Autodesk Fusion 360 part; units mm, degrees
(part 2 of 3)
  point P10 (75, -26)
  point P11 (105, -26)
  point P12 (60, 0)
  point P13 (60, 0)
  point P14 (90, 0)
  point P15 (60, 0)
  point P16 (90, 0)
  point P17 (15, -26)
  point P18 (15, -26)
  point P19 (45, -26)
  point P20 (15, -26)
  point P21 (45, -26)
  point P22 (105, -26)
  point P23 (60, 0)
  point P24 (105, -26)
  point P25 (90, 0)
  point P26 (90, 0)
  point P27 (60, 0)
  point P28 (75, -26)
  point P29 (75, -26)
  point P30 (75, -26)
  point P31 (60, 0)
  point P32 (30, 0)
  point P33 (30, 0)
  point P34 (60, -52)
  point P35 (75, -78)
  point P36 (60, -52)
  point P37 (90, -52)
  point P38 (90, -52)
  point P39 (75, -78)
  point P40 (60, -52)
  point P41 (0, -52)
  point P42 (105, -78)
  point P43 (30, -52)
  point P44 (75, -78)
  point P45 (0, -52)
  point P46 (105, -78)
  point P47 (0, -52)
  point P48 (15, -78)
  point P49 (45, -78)
  point P50 (15, -78)
  point P51 (15, -78)
  point P52 (45, -78)
  point P53 (15, -78)
  point P54 (15, -78)
  point P55 (45, -78)
  point P56 (15, -78)
  point P57 (45, -78)
  point P58 (105, -78)
  point P59 (60, -52)
  point P60 (105, -78)
  point P61 (90, -52)
  point P62 (90, -52)
  point P63 (60, -52)
  point P64 (75, -78)
  point P65 (75, -78)
  point P66 (75, -78)
  point P67 (60, -52)
  point P68 (0, -52)
  point P69 (0, -52)
  point P70 (30, -52)
  point P71 (30, -52)
  point P72 (0, -52)
  point P73 (30, -52)
  dimension "d7" = 16
  dimension "d8" = 16
  dimension "d9" = 2
  dimension "d10" = 14.5
  dimension "d11" = 14.5
  dimension "d14" = 16
  dimension "d15" = 16
  dimension "d16" = 2
  dimension "d17" = 14.5
  dimension "d18" = 14.5
  dimension "d19" = 16
  dimension "d20" = 16
  dimension "d21" = 2
  dimension "d22" = 14.5
  dimension "d23" = 14.5
  dimension "d24" = 16
  dimension "d25" = 16
  dimension "d26" = 2
  dimension "d27" = 14.5
  dimension "d28" = 14.5
  dimension "d29" = 16
  dimension "d30" = 16
  dimension "d31" = 2
  dimension "d32" = 14.5
  dimension "d33" = 14.5
  dimension "d34" = 16
  dimension "d35" = 16
  dimension "d36" = 2
  dimension "d37" = 14.5
  dimension "d38" = 14.5
  dimension "d39" = 16
  dimension "d40" = 16
  dimension "d41" = 2
  dimension "d42" = 14.5
  dimension "d43" = 14.5
  dimension "d44" = 16
  dimension "d45" = 16
  dimension "d46" = 2
  dimension "d47" = 14.5
  dimension "d48" = 14.5
  dimension "d49" = 16
  dimension "d50" = 16
  dimension "d51" = 2
  dimension "d52" = 14.5
  dimension "d53" = 14.5
  dimension "d54" = 16
  dimension "d55" = 16
  dimension "d56" = 2
  dimension "d57" = 14.5
  dimension "d58" = 14.5
  dimension "d59" = 16
  dimension "d60" = 16
  dimension "d61" = 2
  dimension "d62" = 14.5
  dimension "d63" = 14.5
  dimension "d64" = 16
  dimension "d65" = 16
  dimension "d66" = 2
  dimension "d67" = 14.5
  dimension "d68" = 14.5
  dimension "d69" = 16
  dimension "d70" = 16
  dimension "d71" = 2
  dimension "d72" = 14.5
  dimension "d73" = 14.5
  dimension "d74" = 16
  dimension "d75" = 16
  dimension "d76" = 2
  dimension "d77" = 14.5
  dimension "d78" = 14.5
  dimension "d79" = 16
  dimension "d80" = 16
  dimension "d81" = 2
  dimension "d82" = 14.5
  dimension "d83" = 14.5
  dimension "d84" = 16
  dimension "d85" = 16
  dimension "d86" = 2
  dimension "d87" = 14.5
  dimension "d88" = 14.5
  constraint coincident P33 P32
  constraint coincident P20 P18
  constraint coincident P21 P19
  constraint coincident P31 P27
  constraint coincident P26 P25
  constraint coincident P30 P29
  constraint coincident P24 P22
  constraint coincident P72 P69
  constraint coincident P73 P71
  constraint coincident P56 P54
  constraint coincident P57 P55
  constraint coincident P67 P63
  constraint coincident P62 P61
  constraint coincident P66 P65
  constraint coincident P60 P58
  measures "d7" distance of origin L5
  measures "d8" distance of P33 L11
  measures "d9" distance of L5 L8
  measures "d10" distance of origin L17
  measures "d11" distance of P33 L23
  measures "d14" distance of P20 L47
  measures "d15" distance of P21 L34
  measures "d16" distance of L27 L47
  measures "d17" distance of P20 L45
  measures "d18" distance of P21 L33
  measures "d19" distance of P31 L77
  measures "d20" distance of P26 L78
  measures "d21" distance of L64 L77
  measures "d22" distance of P31 L61
  measures "d23" distance of P26 L93
  measures "d24" distance of P30 L86
  measures "d25" distance of P24 L88
  measures "d26" distance of L81 L86
  measures "d27" distance of P30 L48
  measures "d28" distance of P24 L55
  measures "d29" distance of origin L137
  measures "d30" distance of P33 L115
  measures "d31" distance of L137 L138
  measures "d32" distance of origin L126
  measures "d33" distance of P33 L116
  measures "d34" distance of P20 L124
  measures "d35" distance of P21 L127
  measures "d36" distance of L124 L140
  measures "d37" distance of P20 L155
  measures "d38" distance of P21 L120
  measures "d39" distance of P31 L185
  measures "d40" distance of P26 L175
  measures "d41" distance of L185 L191
  measures "d42" distance of P31 L170
  measures "d43" distance of P26 L99
  measures "d44" distance of P30 L150
  measures "d45" distance of P24 L147
  measures "d46" distance of L150 L163
  measures "d47" distance of P30 L158
  measures "d48" distance of P24 L151
  measures "d49" distance of P72 L360
  measures "d50" distance of P73 L338
  measures "d51" distance of L309 L360
  measures "d52" distance of P72 L381
  measures "d53" distance of P73 L340
  measures "d54" distance of P56 L319
  measures "d55" distance of P57 L327
  measures "d56" distance of L319 L332
  measures "d57" distance of P56 L275
  measures "d58" distance of P57 L331
  measures "d59" distance of P67 L365
  measures "d60" distance of P62 L375
  measures "d61" distance of L342 L365
  measures "d62" distance of P67 L336
  measures "d63" distance of P62 L352
  measures "d64" distance of P66 L300
  measures "d65" distance of P60 L320
  measures "d66" distance of L274 L300
  measures "d67" distance of P66 L203
  measures "d68" distance of P60 L317
  measures "d69" distance of P72 L369
  measures "d70" distance of P73 L263
  measures "d71" distance of L369 L379
  measures "d72" distance of P72 L358
  measures "d73" distance of P73 L228
  measures "d74" distance of P56 L196
  measures "d75" distance of P57 L214
  measures "d76" distance of L196 L334
  measures "d77" distance of P56 L219
  measures "d78" distance of P57 L292
  measures "d79" distance of P67 L246
  measures "d80" distance of P62 L235
  measures "d81" distance of L221 L246
  measures "d82" distance of P67 L222
  measures "d83" distance of P62 L227
  measures "d84" distance of P66 L212
  measures "d85" distance of P60 L199
  measures "d86" distance of L208 L212
  measures "d87" distance of P66 L205
  measures "d88" distance of P60 L201
extrude "Extrude2" add sketch "Sketch1" along normal blind 100 contours L0 L5 L7 L8 L12 L17 L19 L20 L37 L43 L96 L118 L126 L128 L129 L137 L138 L143 L145 L161 | L0 L5 L6 L7 L18 L19 L74 L94 L96 L101 L107 L118 L129 L133 L137 L181 | L0 L1 L2 L3 L7 L8 L12 L13 L14 L15 L28 L37 L96 L102 L104 L105 L109 L111 L112 L118 L138 L143 L145 L169 | L6 L11 L50 L59 L64 L67 L74 L80 L106 L107 L115 L136 L176 L181 L187 L191 | L6 L11 L18 L23 L31 L38 L59 L65 L74 L94 L101 L107 L115 L116 L130 L133 L136 L139 L179 L181 | L4 L5 L21 L27 L30 L38 L97 L131 L137 L139 L140 L162 | L4 L5 L8 L9 L16 L17 L20 L21 L24 L30 L37 L43 L97 L98 L126 L128 L131 L137 L138 L142 L145 L161 L162 L168 | L9 L10 L21 L22 L27 L30 L35 L38 L42 L43 L45 L47 L117 L119 L124 L128 L131 L139 L140 L141 L142 L148 L155 L162 | L22 L35 L43 L47 L60 L94 L101 L117 L119 L124 L128 L189 | L3 L4 L8 L9 L15 L16 L24 L28 L37 L41 L97 L98 L102 L109 L111 L114 L138 L142 L145 L168 | L3 L4 L28 L41 L97 L102 L111 L114 L237 L265 L266 L345 | L50 L56 L67 L71 L73 L75 L77 L78 L79 L93 L99 L106 L167 L171 L174 L175 L176 L180 L184 L185 | L50 L61 L64 L67 L68 L75 L77 L80 L84 L87 L106 L170 L171 L172 L176 L177 L185 L187 L190 L191 | L10 L11 L22 L23 L25 L31 L35 L38 L60 L65 L92 L94 L101 L115 L116 L117 L119 L123 L130 L139 L141 L179 L183 L189 | L28 L39 L41 L46 L111 L114 L144 L146 L225 L234 L237 L242 L265 L266 L271 L280 L288 L309 L345 L379 | L28 L39 L111 L146 L192 L240 L241 L242 L244 L247 L249 L258 L260 L261 L264 L266 L270 L271 L345 L355 | L10 L11 L25 L66 L87 L92 L115 L123 L141 L153 L183 L190 | L25 L31 L33 L34 L49 L52 L60 L66 L82 L87 L92 L95 L103 L113 L120 L123 L127 L130 L134 L153 L173 L183 L189 L190 | L31 L34 L52 L62 L64 L95 L113 L127 L130 L173 L188 L191 | L56 L57 L58 L71 L72 L76 L78 L84 L86 L93 L99 L100 L110 L150 L174 L175 L177 L178 L180 L186 | L55 L56 L63 L72 L76 L78 L83 L88 L100 L147 L149 L151 L164 L174 L175 L186 L230 L235 L375 L380 | L9 L10 L42 L45 L141 L142 L148 L155 L280 L288 L324 L326 | L198 L204 L218 L220 L224 L226 L238 L241 L245 L247 L252 L254 L260 L264 L269 L290 L299 L301 L332 L334 | L192 L223 L226 L229 L231 L240 L241 L244 L245 L247 L254 L257 L260 L261 L264 L268 L269 L285 L309 L379 | L49 L52 L61 L62 L64 L68 L70 L77 L84 L87 L90 L95 L103 L108 L113 L170 L172 L173 L177 L182 L185 L188 L190 L191 | L49 L70 L71 L77 L81 L90 L103 L108 L163 L180 L182 L185 | L26 L27 L29 L36 L42 L44 L45 L47 L124 L125 L132 L140 L148 L154 L155 L156 L278 L280 L281 L287 L288 L308 L324 L326 | L26 L27 L29 L125 L140 L156 L237 L265 L278 L308 L360 L369 | L36 L44 L47 L124 L132 L154 L248 L267 L281 L287 L339 L362 | L26 L39 L44 L46 L125 L132 L144 L146 L225 L234 L237 L265 L278 L280 L288 L308 L309 L312 L356 L358 L360 L369 L379 L381 | L39 L44 L132 L146 L192 L244 L312 L323 L350 L356 L358 L381 | L48 L57 L58 L62 L70 L71 L76 L81 L84 L85 L86 L90 L100 L108 L110 L150 L158 L163 L165 L177 L178 L180 L182 L188 | L33 L49 L60 L82 L103 L120 L134 L189 L239 L267 L339 L354 | L29 L32 L36 L40 L121 L135 L154 L156 L228 L233 L248 L253 L263 L267 L281 L287 L324 L326 L338 L339 L340 L341 L362 L378 | L32 L51 L66 L121 L153 L160 L253 L263 L324 L326 L338 L341 | L192 L223 L226 L229 L231 L244 L245 L257 L268 L279 L285 L305 L309 L312 L323 L350 L356 L358 L360 L369 L370 L371 L379 L381 | L63 L91 L122 L164 L227 L235 L293 L313 L344 L347 L352 L375 | L53 L63 L69 L83 L86 L91 L122 L149 L150 L152 L157 L164 L227 L230 L235 L255 L352 L375 L377 L380 | L32 L33 L34 L40 L51 L66 L82 L89 L120 L121 L127 L134 L135 L153 L160 L166 L239 L251 L253 L267 L339 L341 L354 L374 | L196 L197 L198 L202 L204 L218 L219 L268 L275 L285 L289 L290 L291 L299 L301 L319 L321 L332 L334 L364 | L193 L196 L198 L200 L202 L204 L215 L273 L282 L283 L290 L291 L301 L319 L325 L328 | L195 L199 L201 L206 L207 L210 L211 L212 L213 L216 L235 L286 L293 L300 L303 L316 L317 L320 L335 L344 L349 L351 L353 L375 | L212 L227 L235 L293 L295 L300 L313 L316 L318 L329 L343 L344 L347 L349 L351 L352 L353 L359 L363 L375 | L48 L62 L76 L85 L100 L158 L165 L188 L230 L236 L346 L380 | L226 L245 L262 L279 L296 L305 L332 L334 L360 L369 L370 L371 | L34 L40 L89 L127 L135 L166 L221 L236 L251 L342 L346 L374 | L48 L53 L54 L69 L81 L85 L86 L91 L122 L150 L152 L157 L158 L159 L163 L165 L230 L232 L236 L255 L346 L357 L377 L380 | L193 L200 L209 L214 L215 L272 L273 L276 L282 L283 L292 L302 L314 L315 L325 L327 L328 L331 L348 L373 | L200 L206 L207 L208 L214 L216 L217 L273 L274 L282 L304 L314 L315 L325 L327 L335 | L196 L197 L219 L259 L262 L268 L275 L279 L285 L289 L296 L305 L307 L310 L319 L321 L323 L332 L334 L350 L361 L364 L370 L371 | L51 L53 L54 L89 L157 L159 L160 L166 L221 L222 L232 L236 L239 L246 L251 L336 L337 L342 L346 L354 L357 L365 L374 L383 | L54 L81 L91 L122 L159 L163 L232 L239 L246 L354 L357 L365 | L29 L40 L135 L156 L228 L233 L262 L294 L296 L340 L372 L378 | L228 L233 L248 L256 L259 L262 L263 L272 L277 L294 L296 L298 L307 L310 L321 L338 L340 L361 L362 L364 L368 L372 L373 L378 | L196 L248 L259 L272 L307 L310 L319 L323 L350 L361 L362 L373 | L193 L250 L256 L263 L277 L283 L298 L306 L321 L338 L364 L368 | L194 L203 L205 L206 L207 L208 L210 L212 L213 L216 L217 L243 L274 L300 L304 L311 L333 L335 L351 L353 | L51 L53 L157 L160 L222 L250 L306 L318 L336 L337 L343 L383 | L194 L203 L205 L208 L212 L243 L274 L295 L297 L300 L311 L313 L318 L322 L329 L333 L343 L347 L351 L353 L359 L363 L366 L376 | L208 L246 L274 L276 L297 L313 L322 L347 L348 L365 L366 L376 | L193 L209 L214 L250 L256 L272 L276 L277 L283 L284 L292 L294 L298 L302 L306 L327 L330 L331 L348 L367 L368 L372 L373 L382 | L214 L221 L243 L284 L294 L311 L327 L330 L342 L367 L372 L382 | L221 L222 L243 L246 L250 L276 L284 L297 L306 L311 L318 L322 L330 L336 L337 L342 L343 L348 L365 L366 L367 L376 L382 L383
extrude "Extrude3" add sketch "Sketch1" along normal blind 3
sketch "Sketch2" plane through (0, 0, 0) normal (1, 0, 0) x (0, 0, -1)
  circle A0 centre (0, 0) radius 100.9277
  line L0 (0, 100.9277) -> (-120.0555, 100.9277)
  line L1 (-100.9261, -0.5759) -> (-100.9261, 117.8677)
  constraint coincident A0.centre origin
  constraint coincident A0 L0.start
  constraint tangent A0 L0
  constraint horizontal L0
  constraint coincident A0 L1.start
  constraint perpendicular L0 L1
extrude "Extrude4" cut sketch "Sketch2" along normal blind 169 and the other way blind 53 contours A0 L0 L1
sketch "Sketch3" plane through (0, 0, 0) normal (0, 1, 0) x (1, 0, 0)
  circle A0 centre (0, 0) radius 1.5
  circle A1 centre (30, 0) radius 1.5
  circle A2 centre (15, -26) radius 1.5
  circle A3 centre (0, -52) radius 1.5
  circle A4 centre (15, -78) radius 1.5
  circle A5 centre (45, -78) radius 1.5
  circle A6 centre (30, -52) radius 1.5
  circle A7 centre (45, -26) radius 1.5
  circle A8 centre (60, 0) radius 1.5
  circle A9 centre (90, 0) radius 1.5
  circle A10 centre (105, -26) radius 1.5
  circle A11 centre (75, -26) radius 1.5
  circle A12 centre (60, -52) radius 1.5
  circle A13 centre (75, -78) radius 1.5
  circle A14 centre (105, -78) radius 1.5
  circle A15 centre (90, -52) radius 1.5
  point P0 (15, -78)
  point P1 (0, -52)
  point P2 (30, -52)
  point P3 (15, -26)
  point P4 (30, 0)
  point P5 (45, -26)
  point P6 (60, 0)
  point P7 (90, 0)
  point P8 (75, -26)
  point P9 (105, -26)
  point P10 (90, -52)
  point P11 (60, -52)
  point P12 (45, -78)
  point P13 (75, -78)
  point P14 (105, -78)
  dimension "d97" = 3
  constraint coincident A0.centre origin
  constraint coincident P4 A1.centre
  constraint coincident P3 A2.centre
  constraint coincident P1 A3.centre
  constraint coincident P0 A4.centre
  constraint coincident P12 A5.centre
  constraint coincident P2 A6.centre
  constraint coincident P5 A7.centre
  constraint coincident P6 A8.centre
  constraint coincident P7 A9.centre
  constraint coincident P9 A10.centre
  constraint coincident P8 A11.centre
  constraint coincident P11 A12.centre
  constraint coincident P13 A13.centre
  constraint coincident P14 A14.centre
  constraint coincident P10 A15.centre
  constraint equal A4 A5
  constraint equal A5 A13
  constraint equal A13 A14
  constraint equal A3 A14
  constraint equal A3 A6
  constraint equal A6 A12
  constraint equal A12 A15
  constraint equal A2 A15
  constraint equal A2 A7
  constraint equal A7 A11
  constraint equal A10 A11
  constraint equal A0 A10
  constraint equal A0 A1
  constraint equal A1 A8
  constraint equal A8 A9
  measures "d97" diameter of A0
equation "d7 = size1"
equation "d8 = size1"
equation "d10 = size2"
equation "d11 = size2"
equation "d14 = size1"
equation "d17 = size2"
equation "d18 = size2"
equation "d19 = size1"
equation "d20 = size1"
equation "d22 = size2"
equation "d23 = size2"
equation "d24 = size1"
equation "d25 = size1"
equation "d27 = size2"
equation "d28 = size2"
equation "d29 = size1"
equation "d30 = size1"
equation "d32 = size2"
equation "d33 = size2"
equation "d34 = size1"
equation "d37 = size2"
equation "d38 = size2"
equation "d39 = size1"
equation "d40 = size1"
equation "d42 = size2"
equation "d43 = size2"
equation "d44 = size1"
equation "d45 = size1"
equation "d47 = size2"
equation "d48 = size2"
equation "d49 = size1"
equation "d50 = size1"
equation "d52 = size2"
equation "d53 = size2"
equation "d54 = size1"
equation "d55 = size1"
equation "d57 = size2"
equation "d58 = size2"
equation "d59 = size1"
equation "d60 = size1"
equation "d62 = size2"
equation "d63 = size2"
equation "d64 = size1"
equation "d65 = size1"
equation "d67 = size2"
equation "d68 = size2"
equation "d69 = size1"
equation "d70 = size1"
equation "d72 = size2"
equation "d73 = size2"
equation "d74 = size1"
equation "d77 = size2"
equation "d78 = size2"
equation "d79 = size1"
equation "d80 = size1"
equation "d82 = size2"
equation "d83 = size2"
equation "d84 = size1"
equation "d85 = size1"
equation "d87 = size2"
equation "d88 = size2"
equation "size1 = 16 mm"
equation "size2 = 14.5 mm"

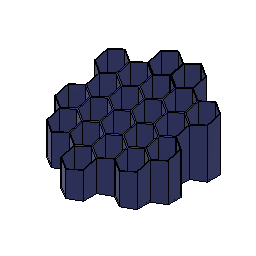
design "hexagon-06"
Autodesk Fusion 360 part; units mm, degrees
sketch "Sketch1" plane through (0, 0, 0) normal (0, 1, 0) x (1, 0, 0)
  line L0 (15.0321, 8.6045) -> (0.0644, 17.3204)
  line L1 (0.0644, 17.3204) -> (-14.9677, 8.7159)
  line L2 (-14.9677, 8.7159) -> (-15.0321, -8.6045)
  line L3 (-15.0321, -8.6045) -> (-0.0644, -17.3204)
  line L4 (-0.0644, -17.3204) -> (14.9677, -8.7159)
  line L5 (14.9677, -8.7159) -> (15.0321, 8.6045)
  line L6 (14.9677, -8.7159) -> (-0.0644, -17.3204)
  line L7 (-0.0644, -17.3204) -> (-0.1287, -34.6408)
  line L8 (-0.1287, -34.6408) -> (14.839, -43.3567)
  line L9 (14.839, -43.3567) -> (29.8711, -34.7523)
  line L10 (29.8711, -34.7523) -> (29.9354, -17.4319)
  line L11 (29.9354, -17.4319) -> (14.9677, -8.7159)
  line L12 (14.839, -43.3567) -> (-0.1287, -34.6408)
  line L13 (-0.1287, -34.6408) -> (-15.1608, -43.2452)
  line L14 (-15.1608, -43.2452) -> (-15.2252, -60.5656)
  line L15 (-15.2252, -60.5656) -> (-0.2575, -69.2816)
  line L16 (-0.2575, -69.2816) -> (14.7746, -60.6771)
  line L17 (14.7746, -60.6771) -> (14.839, -43.3567)
  line L18 (14.2, 8.1984) -> (0, 16.3967)
  line L19 (0, 16.3967) -> (-14.2, 8.1984)
  line L20 (-14.2, 8.1984) -> (-14.2, -8.1984)
  line L21 (-14.2, -8.1984) -> (0, -16.3967)
  line L22 (0, -16.3967) -> (14.2, -8.1984)
  line L23 (14.2, -8.1984) -> (14.2, 8.1984)
  line L24 (29.1033, -17.838) -> (14.9033, -9.6396)
  line L25 (14.9033, -9.6396) -> (0.7033, -17.838)
  line L26 (0.7033, -17.838) -> (0.7033, -34.2347)
  line L27 (0.7033, -34.2347) -> (14.9033, -42.4331)
  line L28 (14.9033, -42.4331) -> (29.1033, -34.2347)
  line L29 (29.1033, -34.2347) -> (29.1033, -17.838)
  line L30 (14.0069, -43.7628) -> (-0.1931, -35.5644)
  line L31 (-0.1931, -35.5644) -> (-14.3931, -43.7628)
  line L32 (-14.3931, -43.7628) -> (-14.3931, -60.1595)
  line L33 (-14.3931, -60.1595) -> (-0.1931, -68.3579)
  line L34 (-0.1931, -68.3579) -> (14.0069, -60.1595)
  line L35 (14.0069, -60.1595) -> (14.0069, -43.7628)
  line L36 (14.7746, -60.6771) -> (-0.2575, -69.2816)
  line L37 (-0.2575, -69.2816) -> (-0.3218, -86.6019)
  line L38 (-0.3218, -86.6019) -> (14.6459, -95.3179)
  line L39 (14.6459, -95.3179) -> (29.678, -86.7134)
  line L40 (29.678, -86.7134) -> (29.7423, -69.393)
  line L41 (29.7423, -69.393) -> (14.7746, -60.6771)
  line L42 (28.9103, -69.7991) -> (14.7103, -61.6007)
  line L43 (14.7103, -61.6007) -> (0.5103, -69.7991)
  line L44 (0.5103, -69.7991) -> (0.5103, -86.1959)
  line L45 (0.5103, -86.1959) -> (14.7103, -94.3942)
  line L46 (14.7103, -94.3942) -> (28.9103, -86.1959)
  line L47 (28.9103, -86.1959) -> (28.9103, -69.7991)
  line L48 (44.7746, -60.6771) -> (29.7425, -69.2816)
  line L49 (44.9677, -8.7159) -> (45.0321, 8.6045)
  line L50 (44.9033, -9.6396) -> (30.7033, -17.838)
  line L51 (29.9356, -17.3204) -> (44.9677, -8.7159)
  line L52 (15.8, 8.1984) -> (15.8, -8.1984)
  line L53 (14.7748, -60.5656) -> (29.7425, -69.2816)
  line L54 (30, -16.3967) -> (44.2, -8.1984)
  line L55 (29.7425, -69.2816) -> (29.6782, -86.6019)
  line L56 (44.7103, -61.6007) -> (30.5103, -69.7991)
  line L57 (29.8069, -68.3579) -> (44.0069, -60.1595)
  line L58 (45.0321, 8.6045) -> (30.0644, 17.3204)
  line L59 (15.0323, 8.7159) -> (14.9679, -8.6045)
  line L60 (30.5103, -69.7991) -> (30.5103, -86.1959)
  line L61 (30.7033, -17.838) -> (30.7033, -34.2347)
  line L62 (29.8713, -34.6408) -> (14.8392, -43.2452)
  line L63 (15.8, -8.1984) -> (30, -16.3967)
  line L64 (30, 16.3967) -> (15.8, 8.1984)
  line L65 (29.8069, -35.5644) -> (15.6069, -43.7628)
  line L66 (44.839, -43.3567) -> (29.8713, -34.6408)
  line L67 (30.0644, 17.3204) -> (15.0323, 8.7159)
  line L68 (44.0069, -43.7628) -> (29.8069, -35.5644)
  line L69 (29.9356, -17.3204) -> (29.8713, -34.6408)
  line L70 (44.2, -8.1984) -> (44.2, 8.1984)
  line L71 (30.7033, -34.2347) -> (44.9033, -42.4331)
  line L72 (44.9677, -8.7159) -> (29.9356, -17.3204)
  line L73 (44.2, 8.1984) -> (30, 16.3967)
  line L74 (58.9103, -69.7991) -> (44.7103, -61.6007)
  line L75 (59.9354, -17.4319) -> (44.9677, -8.7159)
  line L76 (59.7423, -69.393) -> (44.7746, -60.6771)
  line L77 (44.9033, -42.4331) -> (59.1033, -34.2347)
  line L78 (59.678, -86.7134) -> (59.7423, -69.393)
  line L79 (59.1033, -17.838) -> (44.9033, -9.6396)
  line L80 (44.6459, -95.3179) -> (59.678, -86.7134)
  line L81 (44.839, -43.3567) -> (59.8711, -34.7523)
  line L82 (59.8711, -34.7523) -> (59.9354, -17.4319)
  line L83 (59.1033, -34.2347) -> (59.1033, -17.838)
  line L84 (15.6069, -60.1595) -> (29.8069, -68.3579)
  line L85 (44.0069, -60.1595) -> (44.0069, -43.7628)
  line L86 (29.6782, -86.6019) -> (44.6459, -95.3179)
  line L87 (30.5103, -86.1959) -> (44.7103, -94.3942)
  line L88 (14.9679, -8.6045) -> (29.9356, -17.3204)
  line L89 (29.7425, -69.2816) -> (44.7746, -60.6771)
  line L90 (29.8713, -34.6408) -> (44.839, -43.3567)
  line L91 (58.9103, -86.1959) -> (58.9103, -69.7991)
  line L92 (44.7103, -94.3942) -> (58.9103, -86.1959)
  line L93 (44.7746, -60.6771) -> (44.839, -43.3567)
  line L94 (14.8392, -43.2452) -> (14.7748, -60.5656)
  line L95 (15.6069, -43.7628) -> (15.6069, -60.1595)
  line L96 (74.7746, -60.6771) -> (59.7425, -69.2816)
  line L97 (74.9677, -8.7159) -> (75.0321, 8.6045)
  line L98 (74.9033, -9.6396) -> (60.7033, -17.838)
  line L99 (59.9356, -17.3204) -> (74.9677, -8.7159)
  line L100 (45.8, 8.1984) -> (45.8, -8.1984)
  line L101 (44.7748, -60.5656) -> (59.7425, -69.2816)
  line L102 (60, -16.3967) -> (74.2, -8.1984)
  line L103 (59.7425, -69.2816) -> (59.6782, -86.6019)
  line L104 (74.7103, -61.6007) -> (60.5103, -69.7991)
  line L105 (59.8069, -68.3579) -> (74.0069, -60.1595)
  line L106 (75.0321, 8.6045) -> (60.0644, 17.3204)
  line L107 (45.0323, 8.7159) -> (44.9679, -8.6045)
  line L108 (60.5103, -69.7991) -> (60.5103, -86.1959)
  line L109 (60.7033, -17.838) -> (60.7033, -34.2347)
  line L110 (59.8713, -34.6408) -> (44.8392, -43.2452)
  line L111 (45.8, -8.1984) -> (60, -16.3967)
  line L112 (60, 16.3967) -> (45.8, 8.1984)
  line L113 (59.8069, -35.5644) -> (45.6069, -43.7628)
  line L114 (74.839, -43.3567) -> (59.8713, -34.6408)
  line L115 (60.0644, 17.3204) -> (45.0323, 8.7159)
  line L116 (74.0069, -43.7628) -> (59.8069, -35.5644)
  line L117 (59.9356, -17.3204) -> (59.8713, -34.6408)
  line L118 (74.2, -8.1984) -> (74.2, 8.1984)
  line L119 (60.7033, -34.2347) -> (74.9033, -42.4331)
  line L120 (74.9677, -8.7159) -> (59.9356, -17.3204)
  line L121 (74.2, 8.1984) -> (60, 16.3967)
  line L122 (88.9103, -69.7991) -> (74.7103, -61.6007)
  line L123 (89.9354, -17.4319) -> (74.9677, -8.7159)
  line L124 (89.7423, -69.393) -> (74.7746, -60.6771)
  line L125 (74.9033, -42.4331) -> (89.1033, -34.2347)
  line L126 (89.678, -86.7134) -> (89.7423, -69.393)
  line L127 (89.1033, -17.838) -> (74.9033, -9.6396)
  line L128 (74.6459, -95.3179) -> (89.678, -86.7134)
  line L129 (74.839, -43.3567) -> (89.8711, -34.7523)
  line L130 (89.8711, -34.7523) -> (89.9354, -17.4319)
  line L131 (89.1033, -34.2347) -> (89.1033, -17.838)
  line L132 (45.6069, -60.1595) -> (59.8069, -68.3579)
  line L133 (74.0069, -60.1595) -> (74.0069, -43.7628)
  line L134 (59.6782, -86.6019) -> (74.6459, -95.3179)
  line L135 (60.5103, -86.1959) -> (74.7103, -94.3942)
  line L136 (44.9679, -8.6045) -> (59.9356, -17.3204)
  line L137 (59.7425, -69.2816) -> (74.7746, -60.6771)
  line L138 (59.8713, -34.6408) -> (74.839, -43.3567)
  line L139 (88.9103, -86.1959) -> (88.9103, -69.7991)
  line L140 (74.7103, -94.3942) -> (88.9103, -86.1959)
  line L141 (74.7746, -60.6771) -> (74.839, -43.3567)
  line L142 (44.8392, -43.2452) -> (44.7748, -60.5656)
  line L143 (45.6069, -43.7628) -> (45.6069, -60.1595)
  line L144 (104.7746, -60.6771) -> (89.7425, -69.2816)
  line L145 (104.9677, -8.7159) -> (105.0321, 8.6045)
  line L146 (104.9033, -9.6396) -> (90.7033, -17.838)
  line L147 (89.9356, -17.3204) -> (104.9677, -8.7159)
  line L148 (75.8, 8.1984) -> (75.8, -8.1984)
  line L149 (74.7748, -60.5656) -> (89.7425, -69.2816)
  line L150 (90, -16.3967) -> (104.2, -8.1984)
  line L151 (89.7425, -69.2816) -> (89.6782, -86.6019)
  line L152 (104.7103, -61.6007) -> (90.5103, -69.7991)
  line L153 (89.8069, -68.3579) -> (104.0069, -60.1595)
  line L154 (105.0321, 8.6045) -> (90.0644, 17.3204)
  line L155 (75.0323, 8.7159) -> (74.9679, -8.6045)
  line L156 (90.5103, -69.7991) -> (90.5103, -86.1959)
  line L157 (90.7033, -17.838) -> (90.7033, -34.2347)
  line L158 (89.8713, -34.6408) -> (74.8392, -43.2452)
  line L159 (75.8, -8.1984) -> (90, -16.3967)
  line L160 (90, 16.3967) -> (75.8, 8.1984)
  line L161 (89.8069, -35.5644) -> (75.6069, -43.7628)
  line L162 (104.839, -43.3567) -> (89.8713, -34.6408)
  line L163 (90.0644, 17.3204) -> (75.0323, 8.7159)
  line L164 (104.0069, -43.7628) -> (89.8069, -35.5644)
  line L165 (89.9356, -17.3204) -> (89.8713, -34.6408)
  line L166 (104.2, -8.1984) -> (104.2, 8.1984)
  line L167 (90.7033, -34.2347) -> (104.9033, -42.4331)
  line L168 (104.9677, -8.7159) -> (89.9356, -17.3204)
  line L169 (104.2, 8.1984) -> (90, 16.3967)
  line L170 (118.9103, -69.7991) -> (104.7103, -61.6007)
  line L171 (119.9354, -17.4319) -> (104.9677, -8.7159)
  line L172 (119.7423, -69.393) -> (104.7746, -60.6771)
  line L173 (104.9033, -42.4331) -> (119.1033, -34.2347)
  line L174 (119.678, -86.7134) -> (119.7423, -69.393)
  line L175 (119.1033, -17.838) -> (104.9033, -9.6396)
  line L176 (104.6459, -95.3179) -> (119.678, -86.7134)
  line L177 (104.839, -43.3567) -> (119.8711, -34.7523)
  line L178 (119.8711, -34.7523) -> (119.9354, -17.4319)
  line L179 (119.1033, -34.2347) -> (119.1033, -17.838)
  line L180 (75.6069, -60.1595) -> (89.8069, -68.3579)
  line L181 (104.0069, -60.1595) -> (104.0069, -43.7628)
  line L182 (89.6782, -86.6019) -> (104.6459, -95.3179)
  line L183 (90.5103, -86.1959) -> (104.7103, -94.3942)
  line L184 (74.9679, -8.6045) -> (89.9356, -17.3204)
  line L185 (89.7425, -69.2816) -> (104.7746, -60.6771)
  line L186 (89.8713, -34.6408) -> (104.839, -43.3567)
  line L187 (118.9103, -86.1959) -> (118.9103, -69.7991)
  line L188 (104.7103, -94.3942) -> (118.9103, -86.1959)
  line L189 (104.7746, -60.6771) -> (104.839, -43.3567)
  line L190 (74.8392, -43.2452) -> (74.7748, -60.5656)
  line L191 (75.6069, -43.7628) -> (75.6069, -60.1595)
  line L192 (30.0644, 17.3204) -> (45.0323, 8.7159)
  line L193 (45.0323, 8.7159) -> (59.9679, 17.3763)
  line L194 (59.9679, 17.3763) -> (59.9356, 34.6411)
  line L195 (59.9356, 34.6411) -> (44.9677, 43.2456)
  line L196 (44.9677, 43.2456) -> (30.0321, 34.5852)
  line L197 (30.0321, 34.5852) -> (30.0644, 17.3204)
  line L198 (59.9679, 17.3763) -> (75.0323, 8.7159)
  line L199 (75.0323, 8.7159) -> (90.0646, 17.4319)
  line L200 (90.0646, 17.4319) -> (90.0325, 34.8082)
  line L201 (90.0325, 34.8082) -> (74.9681, 43.4686)
  line L202 (74.9681, 43.4686) -> (59.9358, 34.7526)
  line L203 (59.9358, 34.7526) -> (59.9679, 17.3763)
  line L204 (104.9677, -8.7159) -> (119.9354, -17.4319)
  line L205 (119.9354, -17.4319) -> (134.9675, -8.8274)
  line L206 (134.9675, -8.8274) -> (135.0319, 8.493)
  line L207 (135.0319, 8.493) -> (120.0642, 17.2089)
  line L208 (120.0642, 17.2089) -> (105.0321, 8.6045)
  line L209 (105.0321, 8.6045) -> (104.9677, -8.7159)
  line L210 (104.839, -43.3567) -> (104.7746, -60.6771)
  line L211 (104.7746, -60.6771) -> (119.7423, -69.393)
  line L212 (119.7423, -69.393) -> (134.7744, -60.7886)
  line L213 (134.7744, -60.7886) -> (134.8388, -43.4682)
  line L214 (134.8388, -43.4682) -> (119.8711, -34.7523)
  line L215 (119.8711, -34.7523) -> (104.839, -43.3567)
  line L216 (44.6459, -95.3179) -> (44.678, -112.6942)
  line L217 (44.678, -112.6942) -> (59.7423, -121.3546)
  line L218 (59.7423, -121.3546) -> (74.7746, -112.6386)
  line L219 (74.7746, -112.6386) -> (74.7425, -95.2623)
  line L220 (74.7425, -95.2623) -> (59.6782, -86.6019)
  line L221 (59.6782, -86.6019) -> (44.6459, -95.3179)
  line L222 (59.2161, 34.1512) -> (45.0323, 42.3775)
  line L223 (45.0323, 42.3775) -> (30.8162, 34.2071)
  line L224 (30.8162, 34.2071) -> (30.7839, 17.8104)
  line L225 (30.7839, 17.8104) -> (44.9677, 9.584)
  line L226 (44.9677, 9.584) -> (59.1838, 17.7544)
  line L227 (59.1838, 17.7544) -> (59.2161, 34.1512)
  line L228 (89.2002, 34.2906) -> (75.0002, 42.489)
  line L229 (75.0002, 42.489) -> (60.8002, 34.2906)
  line L230 (60.8002, 34.2906) -> (60.8002, 17.8939)
  line L231 (60.8002, 17.8939) -> (75.0002, 9.6955)
  line L232 (75.0002, 9.6955) -> (89.2002, 17.8939)
  line L233 (89.2002, 17.8939) -> (89.2002, 34.2906)
  line L234 (134.0371, -43.9271) -> (119.8676, -35.676)
  line L235 (119.8676, -35.676) -> (105.6373, -43.8216)
  line L236 (105.6373, -43.8216) -> (105.5763, -60.2182)
  line L237 (105.5763, -60.2182) -> (119.7458, -68.4693)
  line L238 (119.7458, -68.4693) -> (133.9761, -60.3237)
  line L239 (133.9761, -60.3237) -> (134.0371, -43.9271)
  line L240 (134.2302, 8.0341) -> (120.0607, 16.2852)
  line L241 (120.0607, 16.2852) -> (105.8304, 8.1396)
  line L242 (105.8304, 8.1396) -> (105.7694, -8.257)
  line L243 (105.7694, -8.257) -> (119.9389, -16.5081)
  line L244 (119.9389, -16.5081) -> (134.1692, -8.3626)
  line L245 (134.1692, -8.3626) -> (134.2302, 8.0341)
  line L246 (73.8951, -95.7537) -> (59.68, -87.5815)
  line L247 (59.68, -87.5815) -> (45.4951, -95.8061)
  line L248 (45.4951, -95.8061) -> (45.5254, -112.2028)
  line L249 (45.5254, -112.2028) -> (59.7405, -120.375)
  line L250 (59.7405, -120.375) -> (73.9254, -112.1504)
  line L251 (73.9254, -112.1504) -> (73.8951, -95.7537)
  point P0 (14.9033, -26.0363)
  point P1 (-0.1931, -51.9612)
  point P2 (14.9033, -26.0363)
  point P3 (-0.1931, -51.9612)
  point P4 (14.7103, -77.9975)
  point P5 (14.7103, -77.9975)
  point P6 (44.9033, -26.0363)
  point P7 (29.8069, -51.9612)
  point P8 (44.9033, -26.0363)
  point P9 (30, 0)
  point P10 (30, 0)
  point P11 (29.8069, -51.9612)
  point P12 (44.7103, -77.9975)
  point P13 (30, 0)
  point P14 (44.7103, -77.9975)
  point P15 (74.9033, -26.0363)
  point P16 (59.8069, -51.9612)
  point P17 (74.9033, -26.0363)
  point P18 (60, 0)
  point P19 (60, 0)
  point P20 (59.8069, -51.9612)
  point P21 (74.7103, -77.9975)
  point P22 (60, 0)
  point P23 (74.7103, -77.9975)
  point P24 (104.9033, -26.0363)
  point P25 (89.8069, -51.9612)
  point P26 (104.9033, -26.0363)
  point P27 (90, 0)
  point P28 (90, 0)
  point P29 (89.8069, -51.9612)
  point P30 (104.7103, -77.9975)
  point P31 (90, 0)
  point P32 (104.7103, -77.9975)
  point P33 (59.8713, -34.6408)
  point P34 (45, 25.9808)
  point P35 (75.0002, 26.0922)
  point P36 (119.9998, -0.1115)
  point P37 (119.8067, -52.0726)
  point P38 (59.7103, -103.9783)
  point P39 (45, 25.9808)
  point P40 (75.0002, 26.0922)
  point P41 (119.8067, -52.0726)
  point P42 (119.9998, -0.1115)
  point P43 (59.7103, -103.9783)
  dimension "d29" = 15
  dimension "d30" = 14.2
  dimension "d31" = 14.2
  dimension "d32" = 14.2
  dimension "d33" = 14.2
  dimension "d36" = 90
  dimension "d37" = 0
  dimension "d47" = 14.2
  dimension "d48" = 14.2
  dimension "d49" = 14.2
  dimension "d50" = 14.2
  dimension "d51" = 14.2
  constraint coincident P2 P0
  constraint coincident P3 P1
  constraint coincident P5 P4
  constraint coincident P33 L110.start
  constraint coincident P39 P34
  constraint coincident P40 P35
  constraint coincident P41 P37
  constraint coincident P42 P36
  constraint coincident P43 P38
  measures "d29" distance of origin L5
  measures "d30" distance of origin L23
  measures "d31" distance of P2 L29
  measures "d32" distance of P3 L35
  measures "d33" distance of P5 L47
  measures "d47" distance of P39 L227
  measures "d48" distance of P40 L233
  measures "d49" distance of P41 L239
  measures "d50" distance of P42 L245
  measures "d51" distance of P43 L251
extrude "Extrude2" add sketch "Sketch1" along normal blind 1.6 contours L0 L5 L59 L88 | L0 L5 L49 L51 L58 L59 L67 L72 L88 L107 L136 | L0 L1 L2 L3 L4 L5 L6 L59 L88 | L5 L11 L69 L88 | L4 L6 L7 L8 L11 L12 L62 L69 L94 | L10 L11 L51 L66 L69 L72 L75 L90 L110 L117 L142 | L192 L193 L194 L195 L196 L197 | L10 L11 L66 L69 L90 | L49 L75 L117 L136 | L49 L58 L97 L99 L106 L107 L115 L120 L136 L155 L184 | L49 L58 L107 L136 | L8 L12 L13 L14 L15 L16 L17 L36 L53 L94 | L8 L9 L10 L12 L62 L66 L90 L94 | L75 L82 L99 L114 L117 L120 L123 L138 L158 L165 L190 | L75 L82 L114 L117 L138 | L198 L199 L200 L201 L202 L203 | L8 L12 L17 L53 L94 | L9 L10 L17 L48 L53 L66 L89 L90 L93 L101 L142 | L66 L81 L82 L90 L110 L114 L138 L142 | L97 L106 L145 L147 L154 L155 L163 L168 L184 L209 | L97 L106 L155 L184 | L66 L90 L93 L101 L142 | L97 L123 L165 L184 | L81 L82 L93 L96 L101 L114 L137 L138 L141 L149 L190 | L17 L41 L53 L55 | L16 L36 L37 L38 L39 L40 L41 L55 L86 | L123 L130 L147 L162 L165 L168 L171 L177 L178 L186 L204 L215 | L123 L130 L162 L165 L186 | L114 L129 L130 L138 L158 L162 L186 L190 | L114 L138 L141 L149 L190 | L145 L171 L204 L205 L206 L207 L208 L209 | L40 L41 L48 L55 L76 L86 L89 L103 L221 | L76 L93 L101 L103 | L129 L130 L141 L144 L149 L162 L185 L186 L189 L210 | L40 L41 L55 L86 | L76 L78 L96 L103 L124 L126 L128 L137 L151 L182 L219 L220 | L124 L141 L149 L151 | L76 L78 L103 L134 L220 | L172 L177 L189 L210 L211 L212 L213 L214 L215 | L124 L126 L144 L151 L172 L174 L176 L182 L185 L211 | L78 L80 L134 L220 L221 | L124 L126 L151 L182 | L78 L80 L128 L134 L216 L217 L218 L219 | L128 L134 L219 L220 | L18 L19 L20 L21 L22 L23 | L24 L25 L26 L27 L28 L29 | L30 L31 L32 L33 L34 L35 | L42 L43 L44 L45 L46 L47 | L50 L61 L71 L77 L79 L83 | L52 L54 L63 L64 L70 L73 | L56 L60 L74 L87 L91 L92 | L57 L65 L68 L84 L85 L95 | L98 L109 L119 L125 L127 L131 | L100 L102 L111 L112 L118 L121 | L104 L108 L122 L135 L139 L140 | L105 L113 L116 L132 L133 L143 | L146 L157 L167 L173 L175 L179 | L148 L150 L159 L160 L166 L169 | L152 L156 L170 L183 L187 L188 | L153 L161 L164 L180 L181 L191 | L222 L223 L224 L225 L226 L227 | L228 L229 L230 L231 L232 L233 | L234 L235 L236 L237 L238 L239 | L240 L241 L242 L243 L244 L245 | L246 L247 L248 L249 L250 L251 makes body 1
extrude "Extrude3" add sketch "Sketch1" along normal blind 80 contours L0 L5 L59 L88 | L0 L5 L49 L51 L58 L59 L67 L72 L88 L107 L136 | L0 L1 L2 L3 L4 L5 L6 L59 L88 | L5 L11 L69 L88 | L4 L6 L7 L8 L11 L12 L62 L69 L94 | L10 L11 L51 L66 L69 L72 L75 L90 L110 L117 L142 | L192 L193 L194 L195 L196 L197 | L10 L11 L66 L69 L90 | L49 L75 L117 L136 | L49 L58 L97 L99 L106 L107 L115 L120 L136 L155 L184 | L49 L58 L107 L136 | L8 L12 L13 L14 L15 L16 L17 L36 L53 L94 | L8 L9 L10 L12 L62 L66 L90 L94 | L75 L82 L99 L114 L117 L120 L123 L138 L158 L165 L190 | L75 L82 L114 L117 L138 | L198 L199 L200 L201 L202 L203 | L8 L12 L17 L53 L94 | L9 L10 L17 L48 L53 L66 L89 L90 L93 L101 L142 | L66 L81 L82 L90 L110 L114 L138 L142 | L97 L106 L145 L147 L154 L155 L163 L168 L184 L209 | L97 L106 L155 L184 | L66 L90 L93 L101 L142 | L97 L123 L165 L184 | L81 L82 L93 L96 L101 L114 L137 L138 L141 L149 L190 | L17 L41 L53 L55 | L16 L36 L37 L38 L39 L40 L41 L55 L86 | L123 L130 L147 L162 L165 L168 L171 L177 L178 L186 L204 L215 | L123 L130 L162 L165 L186 | L114 L129 L130 L138 L158 L162 L186 L190 | L114 L138 L141 L149 L190 | L145 L171 L204 L205 L206 L207 L208 L209 | L40 L41 L48 L55 L76 L86 L89 L103 L221 | L76 L93 L101 L103 | L129 L130 L141 L144 L149 L162 L185 L186 L189 L210 | L40 L41 L55 L86 | L76 L78 L96 L103 L124 L126 L128 L137 L151 L182 L219 L220 | L124 L141 L149 L151 | L76 L78 L103 L134 L220 | L172 L177 L189 L210 L211 L212 L213 L214 L215 | L124 L126 L144 L151 L172 L174 L176 L182 L185 L211 | L78 L80 L134 L220 L221 | L124 L126 L151 L182 | L78 L80 L128 L134 L216 L217 L218 L219 | L128 L134 L219 L220 bodies 1
sketch "Sketch2" plane through (0, 0, 0) normal (1, 0, 0) x (0, 0, -1)
  line L0 (58.2994, 83.577) -> (-124.7141, 32.2408)
  line L1 (-124.7141, 32.2408) -> (-124.7141, 83.577)
  line L2 (-124.7141, 83.577) -> (58.2994, 83.577)
  constraint vertical L1
  constraint perpendicular L1 L2
extrude "Extrude4" cut sketch "Sketch2" along normal blind 159 and the other way blind 41 bodies 1
copy_body "Body->Comp1" bodies 1 removing the originals makes body 2 in component "hexagon-06"
component "hexagon-06" placed x (1, 0, 0) y (0, 1, 0) z (0, 0, 1) at (0, 0, 0)
equation "size1 = 15 mm"
equation "offset1 = 0.8 mm"
equation "d29 = size1"
equation "d30 = size1 - offset1"
equation "d31 = size1 - offset1"
equation "d32 = size1 - offset1"
equation "d33 = size1 - offset1"
equation "d36 = 6 * size1"
equation "d38 = 2 * offset1"
equation "d40 = height"
equation "height = 80 mm"
equation "d47 = size1 - offset1"
equation "d48 = size1 - offset1"
equation "d49 = size1 - offset1"
equation "d50 = size1 - offset1"
equation "d51 = size1 - offset1"

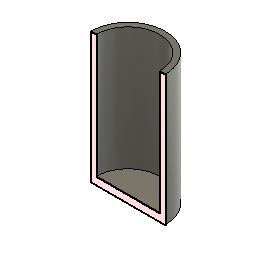
design "tubeToolHolder02"
Autodesk Fusion 360 part; units mm, degrees
sketch "Sketch1" plane through (0, 0, 0) normal (0, 1, 0) x (1, 0, 0)
  circle A0 centre (0, 0) radius 20
  circle A1 centre (0, 0) radius 17
  dimension "d1" = 40
  dimension "d7" = 3
  constraint coincident A0.centre A1.centre
  measures "d1" diameter of A0
  measures "d7" distance of A0 A1
extrude "Extrude1" add sketch "Sketch1" along normal blind 70 makes body 1
extrude "Extrude2" add sketch "Sketch1" along normal blind 4 contours A1 bodies 1
copy_body "Body->Comp1" bodies 1 removing the originals makes body 2 in component "tubeToolHolder02"
component "tubeToolHolder02" placed x (1, 0, 0) y (0, 1, 0) z (0, 0, 1) at (0, 0, 0)

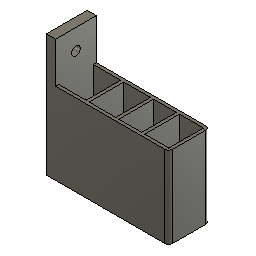
design "item40ToolHolder01"
Autodesk Fusion 360 part; units mm, degrees
sketch "Sketch1" plane through (0, 0, 0) normal (0, 1, 0) x (1, 0, 0)
  line L0 (60, 20) -> (-60, 20)
  line L1 (-60, 20) -> (-60, -20)
  line L2 (-60, -20) -> (60, -20)
  line L3 (60, -20) -> (60, 20)
  line L4 (60, 20) -> (-60, -20) construction
  line L5 (-60, 20) -> (60, -20) construction
  line L6 (57, 17) -> (-57, 17)
  line L7 (-57, 17) -> (-57, -17)
  line L8 (-57, -17) -> (57, -17)
  line L9 (57, -17) -> (57, 17)
  line L10 (57, 17) -> (-57, -17) construction
  line L11 (-57, 17) -> (57, -17) construction
  line L12 (-24.159, 17) -> (-21.159, 17)
  line L13 (-21.159, 17) -> (-21.159, -17)
  line L14 (-21.159, -17) -> (-24.159, -17)
  line L15 (-24.159, -17) -> (-24.159, 17)
  line L16 (8.0431, 17) -> (8.0431, -17)
  line L17 (5.0431, -17) -> (5.0431, 17)
  line L18 (8.0431, -17) -> (5.0431, -17)
  line L19 (5.0431, 17) -> (8.0431, 17)
  line L20 (30.4518, 17) -> (33.4518, 17)
  line L21 (33.4518, 17) -> (33.4518, -17)
  line L22 (30.4518, -17) -> (30.4518, 17)
  line L23 (33.4518, -17) -> (30.4518, -17)
  dimension "d1" = 120
  dimension "d2" = 40
  dimension "d3" = 114
  dimension "d4" = 34
  dimension "d20" = 3
  dimension "d21" = 34
  dimension "d26" = 3
  dimension "d27" = 34
  dimension "d28" = 3
  dimension "d29" = 34
  constraint horizontal L0
  constraint perpendicular L0 L1
  constraint parallel L0 L2
  constraint parallel L1 L3
  constraint coincident L4 origin
  constraint coincident L5 origin
  constraint horizontal L6
  constraint perpendicular L6 L7
  constraint parallel L6 L8
  constraint parallel L7 L9
  constraint coincident L10 origin
  constraint coincident L11 origin
  constraint horizontal L12
  constraint vertical L13
  constraint horizontal L14
  constraint vertical L15
  constraint horizontal L19
  constraint vertical L16
  constraint horizontal L18
  constraint vertical L17
  constraint horizontal L20
  constraint vertical L21
  constraint horizontal L23
  constraint vertical L22
  constraint coincident L6 L12.start
  constraint coincident L6 L17.end
  constraint coincident L6 L20.start
  measures "d1" distance of L1.end L2.end
  measures "d2" distance of L0.end L1.end
  measures "d3" distance of L7.end L8.end
  measures "d4" distance of L6.end L7.end
  measures "d20" distance of L12.start L12.end
  measures "d21" distance of L12.start L14.end
  measures "d26" distance of L17.end L16.start
  measures "d27" distance of L17.start L17.end
  measures "d28" distance of L20.start L20.end
  measures "d29" distance of L22.start L20.start
extrude "Extrude1" add sketch "Sketch1" along normal blind 80 contours L0 L1 L2 L3 | L6 L8 L20 L21 L22 L23 | L6 L8 L16 L17 L18 L19 | L6 L8 L12 L13 L14 L15 makes body 1
extrude "Extrude2" add sketch "Sketch1" along normal blind 4 contours L6 L8 L9 L21 | L6 L8 L20 L21 L22 L23 | L6 L8 L16 L22 | L6 L8 L16 L17 L18 L19 | L6 L8 L13 L17 | L6 L8 L12 L13 L14 L15 | L6 L7 L8 L15 bodies 1
sketch "Sketch2" plane through (0, 0, 0) normal (1, 0, 0) x (0, 0, -1)
  line L0 (-20, 0) -> (20, 0)
  line L1 (20, 0) -> (20, 80)
  line L2 (20, 80) -> (-20, 80)
  line L3 (-20, 80) -> (-20, 0)
  line L4 (20, 120) -> (-20, 120)
  line L5 (-20, 120) -> (-20, 80)
  line L6 (-20, 80) -> (20, 80)
  line L7 (20, 80) -> (20, 120)
  line L8 (20, 120) -> (-20, 80) construction
  line L9 (-20, 120) -> (20, 80) construction
  line L10 (20, 0) -> (-20, 0)
  line L11 (-20, 0) -> (-20, -40)
  line L12 (-20, -40) -> (20, -40)
  line L13 (20, -40) -> (20, 0)
  line L14 (20, 0) -> (-20, -40) construction
  line L15 (-20, 0) -> (20, -40) construction
  circle A0 centre (0, 100) radius 4.25
  circle A1 centre (0, -20) radius 4.25
  point P0 (0, 100)
  point P1 (0, -20)
  dimension "d9" = 40
  dimension "d10" = 40
  dimension "d11" = 40
  dimension "d12" = 40
  dimension "d13" = 8.5
  dimension "d14" = 8.5
  constraint horizontal L4
  constraint perpendicular L4 L5
  constraint parallel L4 L6
  constraint parallel L5 L7
  constraint coincident L8 P0
  constraint coincident L9 P0
  constraint coincident L2.end L3.start
  constraint horizontal L10
  constraint perpendicular L10 L11
  constraint parallel L10 L12
  constraint parallel L11 L13
  constraint coincident L14 P1
  constraint coincident L15 P1
  constraint coincident L0.start L3.end
  constraint coincident P0 A0.centre
  constraint coincident P1 A1.centre
  measures "d9" distance of L2.end L1.end
  measures "d10" distance of L2.end L4.end
  measures "d11" distance of L11.end L12.end
  measures "d12" distance of L0.start L11.end
  measures "d13" diameter of A0
  measures "d14" diameter of A1
extrude "Extrude3" add sketch "Sketch2" along normal blind -60 and the other way blind 51 contours L0 L1 L2 L3 L6 L10 | L2 L4 L5 L6 L7 bodies 1
fillet "Fillet1" radius 4 2 edges at (60, 40, -20) (60, 40, 20) on bodies 1
copy_body "Body->Comp1" bodies 1 removing the originals makes body 2 in component "item40ToolHoplder-01"
component "item40ToolHoplder-01" placed x (1, 0, 0) y (0, 1, 0) z (0, 0, 1) at (0, 0, 0)

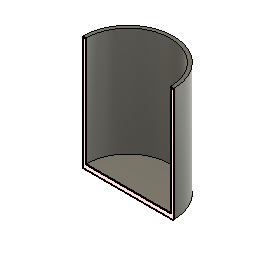
design "tubeToolHolder05"
Autodesk Fusion 360 part; units mm, degrees
sketch "Sketch1" plane through (0, 0, 0) normal (0, 1, 0) x (1, 0, 0)
  circle A0 centre (0, 0) radius 40
  circle A1 centre (0, 0) radius 37
  dimension "d1" = 80
  dimension "d7" = 3
  constraint coincident A0.centre A1.centre
  measures "d1" diameter of A0
  measures "d7" distance of A0 A1
extrude "Extrude1" add sketch "Sketch1" along normal blind 100 makes body 1
extrude "Extrude2" add sketch "Sketch1" along normal blind 4 contours A1 bodies 1
copy_body "Body->Comp1" bodies 1 removing the originals makes body 2 in component "tubeToolHolder05"
component "tubeToolHolder05" placed x (1, 0, 0) y (0, 1, 0) z (0, 0, 1) at (0, 0, 0)

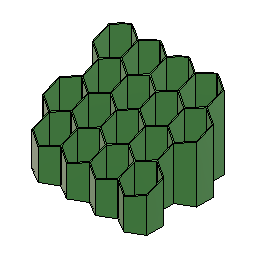
design "hexagon-05"
Autodesk Fusion 360 part; units mm, degrees